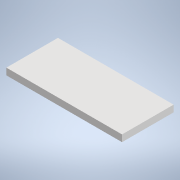
# Autodesk Inventor part: wifi module
Saved by Autodesk Inventor 2022 (Build 260153000, 153)
## iProperties
Created: 2025-01-04
Part Number: wifi module
Material: Типовые
Document SubType Name: Modeling
Designer: akap
Density: 1 g/cm^3
Appearance: По умолчанию
Author: akap
Autodesk Inventor part; units mm, degrees
ref_plane "YZ Plane" through (0, 0, 0) normal (1, 0, 0) x (0, 1, 0)
ref_plane "XZ Plane" through (0, 0, 0) normal (0, 1, 0) x (-1, 0, 0)
ref_plane "XY Plane" through (0, 0, 0) normal (0, 0, 1) x (1, 0, 0)
sketch "Эскиз1" plane through (0, 0, 0) normal (0, 1, 0) x (-1, 0, 0)
  line L0 (-26, 11.6) -> (26, 11.6)
  line L1 (26, 11.6) -> (26, -11.6)
  line L2 (26, -11.6) -> (-26, -11.6)
  line L3 (-26, -11.6) -> (-26, 11.6)
  line L4 (-26, 11.6) -> (26, -11.6) construction
  line L5 (26, 11.6) -> (-26, -11.6) construction
  point P0 (0, 0)
  dimension "d0" = 52
  dimension "d1" = 23.2
  constraints: 12 end point, 2 midpoint, 2 parallel, 1 horizontal, 1 perpendicular
  measures "d0" distance of L1.end L2.end
  measures "d1" distance of L0.end L1.end
extrude "Выдавливание1" add sketch "Эскиз1" along normal blind 3
